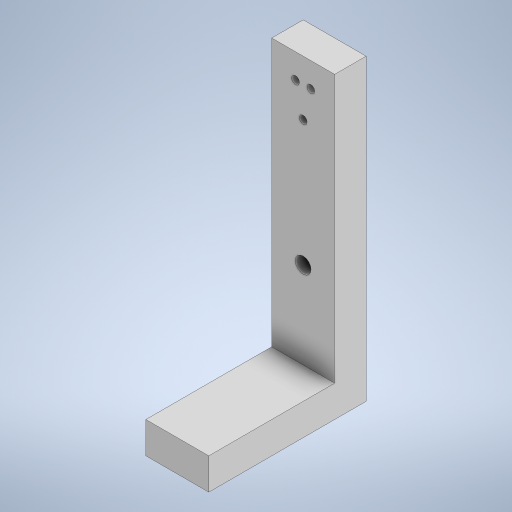
# Autodesk Inventor part: Based
Saved by Autodesk Inventor 2023 (Build 270158000, 158)
## iProperties
Created: 2022-12-28
Part Number: Based
Material: Generic
Document SubType Name: Modeling
Designer: tgr41
Density: 1 g/cm^3
Appearance: Default
Author: tgr41
Autodesk Inventor part; units mm, degrees
ref_plane "YZ Plane" through (0, 0, 0) normal (1, 0, 0) x (0, 1, 0)
ref_plane "XZ Plane" through (0, 0, 0) normal (0, 1, 0) x (-1, 0, 0)
ref_plane "XY Plane" through (0, 0, 0) normal (0, 0, 1) x (1, 0, 0)
sketch "Sketch1" plane through (0, 0, 0) normal (1, 0, 0) x (0, 1, 0)
  line L0 (0, 0) -> (107.95, 0)
  line L1 (107.95, 0) -> (107.95, -12.7)
  line L2 (107.95, -12.7) -> (-12.7, -12.7)
  line L3 (-12.7, -12.7) -> (-12.7, 50.8)
  line L4 (-12.7, 50.8) -> (0, 50.8)
  line L5 (0, 50.8) -> (0, 0)
  dimension "d0" = 107.95
  dimension "d1" = 12.7
  dimension "d2" = 120.65
  dimension "d3" = 63.5
  constraints: 12 end point, 4 perpendicular, 1 horizontal, 1 vertical
  measures "d0" distance of L0.start L0.end
  measures "d1" distance of L0.end L1.end
  measures "d2" distance of L1.end L2.end
  measures "d3" distance of L2.end L3.end
extrude "Extrusion1" add sketch "Sketch1" along normal blind 25.4
sketch "Sketch2" plane through (0, 0, 0) normal (0, 0, 1) x (1, 0, 0)
  line L0 (0, 0) -> (25.4, 0) projected
  circle A0 centre (12.7, 34.925) radius 3.175
  circle A1 centre (12.7, 85.725) radius 1.5875
  circle A2 centre (15.78, 98.0459) radius 1.5875
  line L1 (25.4, 107.95) -> (25.4, 0) projected
  line L2 (0, 107.95) -> (0, 0) projected
  circle A3 centre (9.62, 98.0459) radius 1.5875
  line L3 (0, 107.95) -> (25.4, 107.95) projected
  line L4 (12.7, 107.95) -> (12.7, 0)
  dimension "d7" = 6.35
  dimension "d8" = 3.175
  dimension "d9" = 34.925
  dimension "d10" = 50.8
  dimension "d11" = 3.175
  dimension "d12" = 12.7
  dimension "d17" = 3.175
  dimension "d18" = 12.7
  dimension "d22" = 3.08
  dimension "d23" = 3.08
  constraints: 4 centre point, 2 end point, 2 midpoint
  measures "d7" diameter of A0
  measures "d8" diameter of A1
  measures "d9" distance from line of L0 A0.centre
  measures "d10" distance of A1.centre A0.centre
  measures "d11" diameter of A2
  measures "d12" distance of A2.centre A1.centre
  measures "d17" diameter of A3
  measures "d18" distance of A1.centre A3.centre
  measures "d22" distance from line of L4 A2.centre
  measures "d23" distance from line of A3.centre L4
extrude "Extrusion2" cut sketch "Sketch2" against normal blind 25.4 contours L4 A0 | A0 L4 | L4 A1 | A1 L4 | A2 | A3
body "Solid1"
